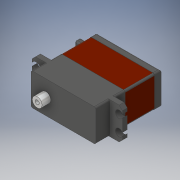
# Autodesk Inventor part: Trackstar_Servo_TS411MG
Saved by Autodesk Inventor 2019 (Build 230136000, 136)
## iProperties
Created: 2020-08-12
Part Number: Trackstar_Servo_TS411MG
Material: Generic
Document SubType Name: Modeling
Designer: Dean.Boonen
Density: 1 g/cm^3
Appearance: Default(1)
Author: Dean.Boonen
Autodesk Inventor part; units mm, degrees
ref_plane "YZ Plane" through (0, 0, 0) normal (1, 0, 0) x (0, 1, 0)
sketch "Sketch1" plane through (0, 0, 0) normal (0, 1, 0) x (-1, 0, 0)
  line L0 (-19.8, -20) -> (19.8, -20)
  line L1 (19.8, -20) -> (19.8, 20)
  line L2 (19.8, 20) -> (-19.8, 20)
  line L3 (-19.8, 20) -> (-19.8, -20)
  line L4 (-19.8, -20) -> (19.8, 20) construction
  line L5 (19.8, -20) -> (-19.8, 20) construction
  point P0 (0, 0)
  dimension "d0" = 39.6
  dimension "d1" = 40
  constraints: 12 end point, 2 midpoint, 2 parallel, 1 horizontal, 1 perpendicular
  measures "d0" distance of L2.end L1.end
  measures "d1" distance of L1.end L0.end
extrude "Extrusion1" add sketch "Sketch1" along normal blind 19.6
sketch "Sketch2" plane through (-19.8, 0, -20) normal (-1, 0, 0) x (0, 0, 1)
  line L0 (31.5, 19.6) -> (28.5, 19.6)
  line L1 (28.5, 19.6) -> (28.5, 0)
  line L2 (28.5, 0) -> (31.5, 0)
  line L3 (31.5, 0) -> (31.5, 19.6)
  line L4 (0, 0) -> (0, 19.6) projected
  line L5 (0, 0) -> (40, 0) projected
  line L6 (0, 19.6) -> (40, 19.6) projected
  point P0 (20, 0)
  dimension "d4" = 28.5
  dimension "d5" = 3
  dimension "d6" = 0
  dimension "d7" = 0
  constraints: 8 end point, 2 parallel, 1 horizontal, 1 perpendicular
  measures "d4" distance between parallel lines of L4 L1
  measures "d5" distance between parallel lines of L1 L3
  measures "d6" distance between parallel lines of L5 L2
  measures "d7" distance between parallel lines of L6 L0
extrude "Extrusion2" add sketch "Sketch2" along normal blind 7.8 contours L3 L2 L1 L0
sketch "Sketch4" plane through (-19.8, 0, 20) normal (0, 0, 1) x (1, 0, 0)
  circle A0 centre (9, 9.8) radius 3
  line L0 (0, 0) -> (39.6, 0) projected
  line L1 (0, 19.6) -> (39.6, 19.6) projected
  circle A1 centre (9, 9.8) radius 1.25
  line L2 (0, 0) -> (0, 19.6) projected
  line L3 (12, 3.6087) -> (12, 15.8306)
  point P0 (19.8, 0)
  dimension "d12" = 9.8
  dimension "d13" = 19.6
  dimension "d14" = 6
  dimension "d15" = 2.5
  dimension "d35" = 9
  dimension "d36" = 12
  constraints: 2 centre point, 2 end point, 1 coincident, 1 vertical
  measures "d12" distance from line of L0 A0.centre
  measures "d13" distance between parallel lines of L1 L0
  measures "d14" diameter of A0
  measures "d15" diameter of A1
  measures "d35" distance from line of L2 A0.centre
  measures "d36" distance between parallel lines of L2 L3
extrude "Extrusion4" add sketch "Sketch4" along normal blind 5.3
ref_plane "Work Plane1" through (19.8, 0, 11.5) normal (0, 0, 1) x (1, 0, 0)
sketch "Sketch5" plane through (19.8, 0, 11.5) normal (0, 0, 1) x (1, 0, 0)
  circle A0 centre (5.2, 5) radius 2.25
  line L0 (-47.4, 0) -> (-47.4, 19.7) projected
  line L1 (6.2685, 9.85) -> (-43.2578, 9.85)
  line L2 (-20.1, 2.75) -> (-20.1, 17.4196)
  circle A1 centre (5.2, 14.7) radius 2.25
  circle A2 centre (-45.4, 5) radius 2.25
  circle A3 centre (-45.4, 14.7) radius 2.25
  line L3 (0, 0) -> (0, 19.6) projected
  line L4 (-39.6, 0) -> (0, 0) projected
  point P0 (-19.8, 0)
  dimension "d18" = 4.5
  dimension "d41" = 5.2
  dimension "d42" = 5
  dimension "d43" = 9.7
  constraints: 4 centre point, 4 end point, 3 symmetric about line, 1 horizontal, 1 vertical, 3 other
  measures "d18" diameter of A0
  measures "d41" distance from line of L3 A0.centre
  measures "d42" distance from line of A0.centre L4
  measures "d43" distance of A0.centre A1.centre
extrude "Extrusion5" cut sketch "Sketch5" against normal blind 5
chamfer "Chamfer1" distance 2 angle 45 2 edges at (-27.6, 19.6, 10) (-27.6, 0, 10)
mirror "Mirror1" about plane through (0, 0, 0) normal (1, 0, 0) of "Extrusion2"
chamfer "Chamfer3" distance 2 angle 45 2 edges at (27.6, 19.6, 10) (27.6, 0, 10)
mirror "Mirror2" about plane through (0, 0, 0) normal (1, 0, 0) of "Extrusion5"
sketch "Sketch7" plane through (-19.8, 0, -20) normal (-1, 0, 0) x (0, 0, 1)
  line L0 (0, 0) -> (0, 19.6) projected
  line L1 (0, 12.1) -> (3.5, 12.1)
  line L2 (3.5, 12.1) -> (3.5, 7.6)
  line L3 (3.5, 7.6) -> (0, 7.6)
  line L4 (0, 7.6) -> (0, 12.1)
  line L5 (0, 0) -> (28.5, 0) projected
  line L6 (28.5, 19.7) -> (0, 19.7) projected
  line L7 (13.8096, 9.85) -> (-5.6461, 9.85) construction
  point P0 (20, 0)
  point P1 (0, 18.7)
  dimension "d44" = 4.5
  dimension "d45" = 19.7
  dimension "d46" = 9.85
  dimension "d47" = 3.5
  constraints: 10 end point, 2 horizontal, 2 parallel, 1 perpendicular, 1 point on line, 1 other
  measures "d44" distance of L1.end L2.end
  measures "d45" distance between parallel lines of L5 L6
  measures "d46" distance between parallel lines of L7 L5
  measures "d47" distance between parallel lines of L0 L2
extrude "Extrusion6" add sketch "Sketch7" along normal blind 10
sketch "Sketch8" plane through (0, 0, 0) normal (0, -1, 0) x (1, 0, 0)
  line L0 (-19.8, 2) -> (19.8, 2)
  line L1 (19.8, 2) -> (19.8, -16)
  line L2 (19.8, -16) -> (-19.8, -16)
  line L3 (-19.8, -16) -> (-19.8, 2)
  line L4 (19.8, -20) -> (-19.8, -20) projected
  line L5 (-19.8, -20) -> (-19.8, 8.5) projected
  line L6 (19.8, 8.5) -> (19.8, -20) projected
  point P0 (0, 0)
  dimension "d52" = 18
  dimension "d55" = 4
  constraints: 8 end point, 2 collinear, 2 parallel, 1 horizontal, 1 perpendicular
  measures "d52" distance between parallel lines of L2 L0
  measures "d55" distance between parallel lines of L2 L4
extrude "Extrusion7" cut sketch "Sketch8" against normal blind 0.1 contours L0 L1 L2 L3
ref_plane "Work Plane2" through (0, 9.8, 0) normal (0, -1, 0) x (1, 0, 0)
mirror "Mirror3" about plane through (0, 9.8, 0) normal (0, -1, 0) of "Extrusion7"
sketch "Sketch9" plane through (-19.8, 0, 8.5) normal (-1, 0, 0) x (0, 0, 1)
  line L0 (-6.5, 19.6) -> (-6.5, 19.5) projected
  line L1 (-24.5, 0.1) -> (-6.5, 0.1) projected
  line L2 (-6.5, 19.5) -> (-24.5, 19.5)
  line L3 (-24.5, 19.5) -> (-24.5, 0.1)
  line L4 (-24.5, 0.1) -> (-6.5, 0.1)
  line L5 (-6.5, 0.1) -> (-6.5, 19.5)
  point P0 (-8.5, 0)
  constraints: 8 end point, 2 parallel, 1 horizontal, 1 perpendicular
extrude "Extrusion8" cut sketch "Sketch9" against normal blind 0.1
mirror "Mirror4" about plane through (0, 0, 0) normal (1, 0, 0) of "Extrusion8"
fillet "Fillet5" radius 1 28 edges at (-19.8, 0, 5.25) (-19.7, 0.1, -7) (-19.8, 0, 15.75) (-19.8, 0, -18) (-19.8, 3.8, -20) (0, 0, -20) (-19.8, 15.85, -20) (-24.8, 12.1, -16.5) (-24.8, 7.6, -16.5) (-24.8, 7.6, -20) (-29.8, 9.85, -20) (-29.8, 12.1, -18.25) (-24.8, 12.1, -20) (-29.8, 9.85, -16.5) (-29.8, 7.6, -18.25) (-19.8, 19.6, -18) (-19.7, 19.5, -7) (-19.8, 19.6, 5.25) (-19.8, 19.6, 15.75) (0, 19.6, -20) (19.8, 19.6, -18) (19.7, 19.5, -7) (19.8, 19.6, 5.25) (19.8, 19.6, 15.75) (19.8, 0, -18) (19.7, 0.1, -7) (19.8, 0, 5.25) (19.8, 0, 15.75)
equation "\"d12\" = 0.5 * d13"
equation "\"d46\" = 0.5 * d45"
body "Solid1"
